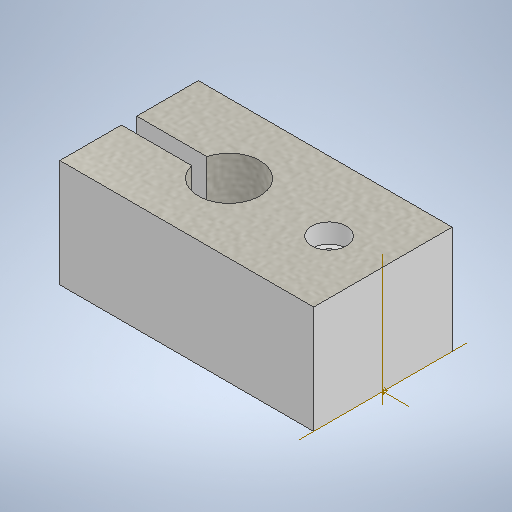
# Autodesk Inventor part: Shaft support
Saved by Autodesk Inventor 2025.2 (Build 292293000, 293)
## iProperties
Created: 2025-01-25
Part Number: Shaft support
Material: Generic
Document SubType Name: Modeling
Designer: caomi
Density: 1 g/cm^3
Appearance: Default
Author: caomi
Autodesk Inventor part; units mm, degrees
ref_plane "YZ Plane" through (0, 0, 0) normal (1, 0, 0) x (0, 1, 0)
ref_plane "XZ Plane" through (0, 0, 0) normal (0, 1, 0) x (-1, 0, 0)
ref_plane "XY Plane" through (0, 0, 0) normal (0, 0, 1) x (1, 0, 0)
sketch "Sketch1" plane through (0, 0, 0) normal (0, 1, 0) x (-1, 0, 0)
  line L0 (16, 0) -> (0, 0)
  line L1 (0, -9) -> (33, -9)
  line L2 (33, -9) -> (33, -1)
  circle A0 centre (20, 0) radius 4
  line L3 (23.873, -1) -> (33, -1)
  line L4 (0, 9) -> (33, 9)
  line L5 (33, 9) -> (33, 1)
  circle A1 centre (20, 0) radius 4
  line L6 (23.873, 1) -> (33, 1)
  line L7 (0, -9) -> (0, 0)
  line L8 (0, 9) -> (0, 0)
  dimension "d2" = 1
  dimension "d3" = 9
  dimension "d4" = 8
  dimension "d27" = 20
  dimension "d28" = 33
  constraints: 18 end point, 4 symmetric about line, 2 horizontal, 2 point on circle, 2 point on line, 1 centre point, 1 line through centre, 1 perpendicular, 1 vertical, 3 other
  measures "d2" distance between parallel lines of L3 L0
  measures "d3" distance between parallel lines of L1 L0
  measures "d4" diameter of A0
  measures "d27" distance from line of L7 A0.centre
  measures "d28" distance between parallel lines of L7 L2
extrude "Extrusion1" add sketch "Sketch1" along normal blind 14 contours A0 L3 L2 L1 L7 L0 | L0 L8 L4 L5 L6 A0
sketch "Sketch7" plane through (0, 14, 0) normal (0, 1, 0) x (1, 0, 0)
  line L0 (0, -9) -> (0, 9) projected
  point P0 (0, 0)
  point P1 (-7, 0)
  point P2 (0, 0)
  dimension "d33" = 7
  constraints: 1 horizontal alignment, 1 midpoint
  measures "d33" distance from line of point (-7, 0) L0
hole "Hole1" at (-7, 14, 0) direction (0, -1, 0) diameter 3 end through all counterbore diameter 4.5 counterbore depth 2.5
sketch "Sketch3" plane through (0, 0, -9) normal (0, 0, -1) x (-1, 0, 0)
  circle A0 centre (28, 7) radius 1.5
  line L0 (33, 0) -> (33, 14) projected
  point P0 (0, 0)
  point P1 (33, 7)
  dimension "d15" = 3
  dimension "d16" = 5
  constraints: 1 centre point, 1 horizontal alignment, 1 midpoint
  measures "d15" diameter of A0
  measures "d16" distance from line of A0.centre L0
sketch "Sketch4" plane through (-33, 0, 9) normal (0, 0, 1) x (1, 0, 0)
  line L0 (6.7898, 10.1) -> (8.5796, 7)
  line L1 (8.5796, 7) -> (6.7898, 3.9)
  line L2 (6.7898, 3.9) -> (3.2102, 3.9)
  line L3 (3.2102, 3.9) -> (1.4204, 7)
  line L4 (1.4204, 7) -> (3.2102, 10.1)
  line L5 (3.2102, 10.1) -> (6.7898, 10.1)
  circle A0 centre (5, 7) radius 1.5 projected
  point P0 (33, 0)
  point P1 (5, 10.1)
  dimension "d20" = 6.2
  constraints: 12 end point, 1 coincident, 1 horizontal, 1 midpoint, 13 other
  measures "d20" distance from line of L2 point (5, 10.1)
sketch "Sketch5" plane through (0, 0, -9) normal (0, 0, -1) x (-1, 0, 0)
  circle A0 centre (28, 7) radius 2.35
  circle A1 centre (28, 7) radius 1.5 projected
  point P0 (0, 0)
  dimension "d23" = 4.7
  constraints: 1 centre point, 1 coincident
  measures "d23" diameter of A0
body "Solid1"
